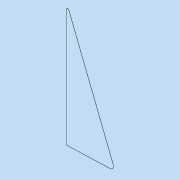
# Autodesk Inventor part: Dây inox
Saved by Autodesk Inventor 2018 (Build 220112000, 112)
## iProperties
Created: 2020-08-11
Part Number: Dây inox
Material: Steel
Document SubType Name: Modeling
Designer: ASUS
Density: 7.85 g/cm^3
Appearance: Plate
Author: ASUS
Autodesk Inventor part; units mm, degrees
ref_plane "YZ Plane" through (0, 0, 0) normal (1, 0, 0) x (0, 1, 0)
ref_plane "XZ Plane" through (0, 0, 0) normal (0, 1, 0) x (-1, 0, 0)
ref_plane "XY Plane" through (0, 0, 0) normal (0, 0, 1) x (1, 0, 0)
sketch "Sketch2" plane through (0, 0, 0) normal (0, 1, 0) x (-1, 0, 0)
  arc A0 (18.5, 0) -> (-17.1894, 6.8392) centre (0, 0) ccw
  arc A1 (-0.6336, -1778.4891) -> (18.5, -1760) centre (0, -1760) ccw
  arc A2 (-690.1687, -1684.5913) -> (-643.1861, -1756.4692) centre (-641.388, -1704) ccw
  line L0 (0, 0) -> (0, -1760)
  line L1 (18.5, 0) -> (18.5, -1760)
  line L2 (-690.1687, -1684.5913) -> (-17.1894, 6.8392)
  line L3 (-0.6336, -1778.4891) -> (-643.1861, -1756.4692)
  dimension "d22" = 37
  dimension "d23" = 37
  dimension "d24" = 105
  dimension "d25" = 56
  dimension "d26" = 1760
  dimension "d27" = 641.388
  constraints: 8 end point, 6 point on circle, 5 tangent, 3 centre point, 2 vertical, 1 coincident
  measures "d22" diameter of A0
  measures "d23" diameter of A1
  measures "d24" diameter of A2
  measures "d25" vertical distance of L0.end A2.centre
  measures "d26" distance of L0.end point (0, 0)
  measures "d27" distance from line of A2.centre L0
sketch "Sketch3" plane through (0, 0, 0) normal (0, 0, 1) x (1, 0, 0)
  circle A0 centre (-18.5, 0) radius 2.5
  point P0 (0, 0)
  dimension "d28" = 5
  constraints: 1 centre point
  measures "d28" diameter of A0
sweep "Sweep1" add profiles "Sketch3" path "Sketch2" path curves L1 A1 L3 A2 L2 A0
body "Solid1"
